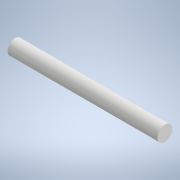
# Autodesk Inventor part: uchwyt1
Saved by Autodesk Inventor 2021 (Build 250183000, 183)
## iProperties
Created: 2021-06-22
Part Number: uchwyt1
Material: Aluminium 3004-O
Document SubType Name: Modeling
Designer: Wojciech Wołczek
Density: 2.71043 g/cm^3
Appearance: Aluminium — polerowane
Author: Wojciech Wołczek
Autodesk Inventor part; units mm, degrees
ref_plane "YZ Plane" through (0, 0, 0) normal (1, 0, 0) x (0, 1, 0)
ref_plane "XZ Plane" through (0, 0, 0) normal (0, 1, 0) x (-1, 0, 0)
ref_plane "XY Plane" through (0, 0, 0) normal (0, 0, 1) x (1, 0, 0)
ref_plane "Płaszczyzna konstrukcyjna1" through (-2.3844, -12.525, -22.8032) normal (1, 0, 0) x (0, 1, 0)
sketch "Szkic1" plane through (-2.3844, -12.525, -22.8032) normal (1, 0, 0) x (0, 1, 0)
  circle A0 centre (0, 0) radius 3
  point P0 (12.525, 22.8032)
  dimension "d0" = 6
  constraints: 1 centre point
  measures "d0" diameter of A0
extrude "Wyciągnięcie proste1" add sketch "Szkic1" along normal blind 60
sketch "Szkic2" plane through (-2.3844, -12.525, -22.8032) normal (-1, 0, 0) x (0, 0, 1)
  line L0 (33, -7.4436) -> (-7, -7.4436)
  line L1 (-7, -7.4436) -> (-7, 7.5564)
  line L2 (-7, 7.5564) -> (33, 7.5564)
  line L3 (33, 7.5564) -> (33, -7.4436)
  line L4 (33, -7.4436) -> (-7, 7.5564) construction
  line L5 (-7, -7.4436) -> (33, 7.5564) construction
  line L6 (0, 16.5188) -> (0, -11.4374)
  circle A0 centre (0, 0) radius 3 projected
  point P0 (22.8032, 12.525)
  point P1 (13, 0.0564)
  dimension "d3" = 40
  dimension "d4" = 15
  dimension "d5" = 7
  constraints: 14 end point, 2 midpoint, 2 parallel, 1 horizontal, 1 perpendicular, 1 vertical, 2 other
  measures "d3" distance of L1.end L2.end
  measures "d4" distance of L0.end L1.end
  measures "d5" distance between parallel lines of L1 L6
extrude "Wyciągnięcie proste2" add sketch "Szkic2" along normal blind 1.5
full round fillet "Zaokrąglenie1" first side at (-2.8844, -19.9687, -16.4698) centre faces at (-2.8844, -9.9687, -29.8032) second side at (-2.8844, -4.9687, -3.1365)
full round fillet "Zaokrąglenie2" first side at (-2.8844, -19.9687, -11.4699) centre faces at (-2.8844, -14.9687, 10.1968) second side at (-2.8844, -4.9687, -0.6365)
